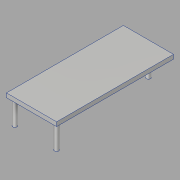
# Autodesk Inventor part: Pi Holder Mk2
Saved by Autodesk Inventor 2017 (Build 210142000, 142)
## iProperties
Created: 2017-01-15
Part Number: Pi Holder Mk2
Material: Aluminum 6061
Document SubType Name: Modeling
Designer: qupec
Density: 2.7 g/cm^3
Appearance: Aluminum - Flat
Author: qupec
Autodesk Inventor part; units mm, degrees
ref_plane "YZ Plane" through (0, 0, 0) normal (1, 0, 0) x (0, 1, 0)
ref_plane "XZ Plane" through (0, 0, 0) normal (0, 1, 0) x (-1, 0, 0)
ref_plane "XY Plane" through (0, 0, 0) normal (0, 0, 1) x (1, 0, 0)
sketch "Sketch1" plane through (0, 0, 0) normal (0, 1, 0) x (-1, 0, 0)
  line L0 (19.05, 44.45) -> (-19.05, 44.45)
  line L1 (-19.05, 44.45) -> (-19.05, -44.45)
  line L2 (-19.05, -44.45) -> (19.05, -44.45)
  line L3 (19.05, -44.45) -> (19.05, 44.45)
  circle A0 centre (11.5, 29) radius 1.375 construction
  circle A1 centre (11.5, -29) radius 1.375 construction
  circle A2 centre (-11.5, 29) radius 1.375 construction
  circle A3 centre (-11.5, -29) radius 1.375 construction
  point P0 (0, 0)
  dimension "d0" = 88.9
  dimension "d1" = 38.1
  dimension "d2" = 19.05
  dimension "d3" = 44.45
  dimension "d4" = 2.75
  dimension "d5" = 2.75
  dimension "d6" = 2.75
  dimension "d7" = 2.75
  dimension "d8" = 58
  dimension "d9" = 58
  dimension "d10" = 23
  dimension "d11" = 11.5
  dimension "d12" = 29
  dimension "d13" = 29
  dimension "d14" = 23
  dimension "d15" = 11.5
  constraints: 8 end point, 4 centre point, 2 parallel, 1 horizontal, 1 perpendicular
  measures "d0" distance of L2.end L0.start
  measures "d1" distance of L0.start L0.end
  measures "d2" distance from line of point (0, 0) L1
  measures "d3" distance from line of point (0, 0) L0
  measures "d4" diameter of A1
  measures "d5" diameter of A0
  measures "d6" diameter of A2
  measures "d7" diameter of A3
  measures "d8" distance of A1.centre A0.centre
  measures "d9" distance of A3.centre A2.centre
  measures "d10" distance of A0.centre A2.centre
  measures "d11" horizontal distance of point (0, 0) A2.centre
  measures "d12" vertical distance of point (0, 0) A0.centre
  measures "d13" vertical distance of point (0, 0) A2.centre
  measures "d14" distance of A1.centre A3.centre
  measures "d15" horizontal distance of point (0, 0) A1.centre
extrude "Extrusion1" add sketch "Sketch1" along normal blind 3.175
sketch "Sketch2" plane through (0, 0, 0) normal (0, -1, 0) x (1, 0, 0)
  circle A0 centre (15.875, 41.275) radius 1.5875
  circle A1 centre (-15.875, 41.275) radius 1.5875
  circle A2 centre (-15.875, -41.275) radius 1.5875
  circle A3 centre (3.175, -41.275) radius 1.5875
  line L0 (-19.05, 44.45) -> (19.05, 44.45) projected
  line L1 (-19.05, -44.45) -> (-19.05, 44.45) projected
  line L2 (19.05, 44.45) -> (19.05, -44.45) projected
  line L3 (19.05, -44.45) -> (-19.05, -44.45) projected
  point P0 (0, 0)
  dimension "d18" = 3.175
  dimension "d19" = 3.175
  dimension "d20" = 3.175
  dimension "d21" = 3.175
  dimension "d22" = 15.875
  dimension "d23" = 3.175
  dimension "d24" = 3.175
  dimension "d25" = 3.175
  dimension "d26" = 3.175
  dimension "d27" = 3.175
  dimension "d28" = 3.175
  dimension "d29" = 3.175
  constraints: 4 centre point
  measures "d18" distance from line of L0 A0.centre
  measures "d19" distance from line of L0 A1.centre
  measures "d20" distance from line of L1 A1.centre
  measures "d21" distance from line of L2 A0.centre
  measures "d22" distance from line of L2 A3.centre
  measures "d23" distance from line of L3 A3.centre
  measures "d24" distance from line of L3 A2.centre
  measures "d25" distance from line of L1 A2.centre
  measures "d26" diameter of A0
  measures "d27" diameter of A1
  measures "d28" diameter of A2
  measures "d29" diameter of A3
extrude "Extrusion2" add sketch "Sketch2" along normal blind 18.415 contours A0 | A1 | A2 | A3
sketch "Sketch3" plane through (0, 3.175, 0) normal (0, 1, 0) x (1, 0, 0)
  circle A0 centre (-14.2875, 17.5562) radius 1.6764
  circle A1 centre (-14.2875, 31.75) radius 1.6764
  line L0 (19.05, -44.45) -> (19.05, 44.45) projected
  line L1 (-19.05, -44.45) -> (19.05, -44.45) projected
  line L2 (-14.2875, 31.75) -> (-14.2875, 17.5562) construction
  line L3 (-19.05, 44.45) -> (-19.05, -44.45) projected
  line L4 (19.05, 44.45) -> (-19.05, 44.45) projected
  point P0 (0, 0)
  dimension "d32" = 3.3528
  dimension "d33" = 3.3528
  dimension "d34" = 14.1938
  dimension "d39" = 4.7625
  dimension "d40" = 12.7
  constraints: 2 centre point, 2 end point, 1 vertical
  measures "d32" diameter of A0
  measures "d33" diameter of A1
  measures "d34" distance of L2.end L2.start
  measures "d39" distance from line of L3 L2.start
  measures "d40" distance from line of L4 L2.start
extrude "Extrusion3" [suppressed]
equation "\"d2\" = 0.5 * d1"
equation "\"d3\" = 0.5 * d0"
equation "\"d5\" = d4"
equation "\"d6\" = d4"
equation "\"d7\" = d4"
equation "\"d9\" = d8"
equation "\"d11\" = 0.5 * d10"
equation "\"d12\" = 0.5 * d8"
equation "\"d13\" = 0.5 * d9"
equation "\"d14\" = d10"
equation "\"d15\" = 0.5 * d14"
equation "\"d19\" = d18"
equation "\"d20\" = d21"
equation "\"d23\" = d18"
equation "\"d24\" = d18"
equation "\"d25\" = d21"
equation "\"d27\" = d26"
equation "\"d28\" = d26"
equation "\"d29\" = d26"
equation "\"d32\" = d33"
body "Solid1"
